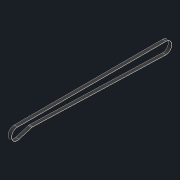
# Autodesk Inventor part: belt_3
Saved by Autodesk Inventor 2021 (Build 250183000, 183)
## iProperties
Created: 2021-07-18
Part Number: belt_3
Material: ゴム
Document SubType Name: Modeling
Designer: yuta0
Density: 0.93 g/cm^3
Appearance: ゴム - 黒
Mass: 6.76349 g
Surface Area: 196.359 cm^2
Volume: 7.27257 cm^3
Author: yuta0
Autodesk Inventor part; units mm, degrees
ref_plane "YZ Plane" through (0, 0, 0) normal (1, 0, 0) x (0, 1, 0)
ref_plane "XZ Plane" through (0, 0, 0) normal (0, 1, 0) x (-1, 0, 0)
ref_plane "XY Plane" through (0, 0, 0) normal (0, 0, 1) x (1, 0, 0)
sketch "スケッチ1" plane through (0, 0, 0) normal (1, 0, 0) x (0, 1, 0)
  arc A0 (17.1887, 0) -> (-16.4352, -5.0335) centre (0, 0) ccw
  arc A1 (-17.18, -439.4511) -> (17.1887, -440) centre (0, -440) ccw
  arc A2 (-4.5853, -45.2689) -> (-4.9501, -42.5346) centre (-13, -45) ccw
  line L0 (-4.9501, -42.5346) -> (-16.4352, -5.0335)
  line L1 (17.1887, -440) -> (17.1887, 0)
  line L2 (-4.5853, -45.2689) -> (-17.18, -439.4511)
  arc A3 (17.6077, 0) -> (-16.8359, -5.1562) centre (0, 0) ccw
  line L3 (-16.8359, -5.1562) -> (-5.3507, -42.6573)
  arc A4 (-5.0041, -45.2555) -> (-5.3507, -42.6573) centre (-13, -45) ccw
  line L4 (-5.0041, -45.2555) -> (-17.5988, -439.4377)
  arc A5 (-17.5988, -439.4377) -> (17.6077, -440) centre (0, -440) ccw
  line L5 (17.6077, -440) -> (17.6077, 0)
  arc A6 (16.8077, 0) -> (-16.0709, -4.9219) centre (0, 0) ccw
  line L6 (-16.0709, -4.9219) -> (-4.5858, -42.423)
  arc A7 (-4.2045, -45.281) -> (-4.5858, -42.423) centre (-13, -45) ccw
  line L7 (-4.2045, -45.281) -> (-16.7992, -439.4632)
  arc A8 (-16.7992, -439.4632) -> (16.8077, -440) centre (0, -440) ccw
  line L8 (16.8077, -440) -> (16.8077, 0)
  dimension "d0" = 34.3775
  dimension "d1" = 34.3775
  dimension "d2" = 440
  dimension "d24" = 0.419
  dimension "d25" = 8
  dimension "d26" = 45
  dimension "d27" = 0.8
  dimension "d29" = 13
  constraints: 18 end point, 18 point on circle, 9 centre point, 6 tangent, 1 coincident, 1 vertical alignment, 10 other
  measures "d0" diameter of A0
  measures "d1" diameter of A1
  measures "d2" distance of A0.centre A1.centre
  measures "d24" distance between parallel lines of L1 L5
  measures "d25" radius of A4
  measures "d26" vertical distance of point (0, 0) A2.centre
  measures "d27" distance between parallel lines of L5 L8
  measures "d29" horizontal distance of point (0, 0) A2.centre
extrude "押し出し1" add sketch "スケッチ1" along normal mid plane 10 contours L1 A1 L2 A2 L0 A0 | L5 A5 L4 A4 L3 A3
